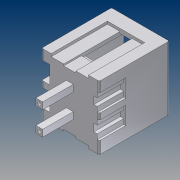
# Autodesk Inventor part: Wago Power In
Saved by Autodesk Inventor 2012 (Build 160160000, 160)
## iProperties
Category: PARTsolutions
Company: Team 801
Created: 2007-11-01
Part Number: Wago Power In
Catalog Web Link: www.team801.org
Description: 734-132 TO 734-154 - HEADER STRAIGHT SOLDER PIN. 1X1 MM / 0.039X 0.039 IN PIN SPACING 3.5 MM / 0.138 IN
Document SubType Name: Modeling
Designer: Jeffrey M
Mass: 0.424756 g
Surface Area: 9.45096 cm^2
Volume: 0.424756 cm^3
Density: 1 g/cm^3
Material: Default
NB: 734-132
NN: 734-132 TO 734-154
NT: HEADER STRAIGHT SOLDER PIN. 1X1 MM / 0.039X 0.039 IN PIN SPACING 3.5 MM / 0.138 IN
NBSYN: $BESTNR.
LINA: 734-132
BESTNR: 734-132
SPANNUNG: 250
BEMESSSTOSSSPG: 3
VERSCHMUTZGRAD: 2
STROM: 10
RM: 3.50
P: 2
HOEHE: 10.30
BREITE: 9.40
TIEFE: 8.50
FARBE: lichtgrau
GEWICHT: 0.602
EAN: 4017332322119
BEMERKUNGEN: L = (No. of poles - 1) x Pin Spacing + 5,9 mm
BOHRLOCHDURCHM: 1,4 +0,1 mm
RGB: 0.82,0.82,0.82,0
KT: DUMMY
PSOL_IDENT_0: {\\partserver001.servicenet\dplatte\cadenas\23d-libs\wago\pg03\serie734\0734-0132_0999-0962.prj},169
PSOL_IDENT_1: {VTYP=3D},{NB=734-132},{LINA=734-132},{NN=734-132 TO 734-154},{DATE=19.07.2007 11:20:09},{GEOMDATE=
PSOL_IDENT_2: 19.07.2007 00:00:00},{VERSION=},{LINEID=220},{LINESUBID=-1},{WBVAR=}  {NB=734-132},{LINA=734-132},{K
PSOL_IDENT_3: T=DUMMY},{BESTNR=734-132},{SPANNUNG=250},{BEMESSSTOSSSPG=3},{VERSCHMUTZGRAD=2},{STROM=10},{RM=3.50},
PSOL_IDENT_4: {P=2},{HOEHE=10.30},{BREITE=9.40},{TIEFE=8.50},{FARBE=lichtgrau},{GEWICHT=0.602},{EAN=4017332322119}
PSOL_IDENT_5: ,{BEMERKUNGEN=L = (No. of poles - 1) x Pin Spacing + 5,9 mm},{BOHRLOCHDURCHM=1,4 +0,1 mm},{RGB=0.82,
PSOL_IDENT_6: 0.82,0.82,0}
Title: Wago Power In
Author: Jeffrey M
Comments: HEADER STRAIGHT SOLDER PIN. 1X1 MM / 0.039X 0.039 IN PIN SPACING 3.5 MM / 0.138 IN
Autodesk Inventor part; units mm, degrees
ref_plane "YZ Plane" through (0, 0, 0) normal (1, 0, 0) x (0, 1, 0)
ref_plane "XZ Plane" through (0, 0, 0) normal (0, 1, 0) x (-1, 0, 0)
ref_plane "XY Plane" through (0, 0, 0) normal (0, 0, 1) x (1, 0, 0)
sketch "Skizze_1" plane through (0, 0, 0) normal (0, 0, 1) x (1, 0, 0)
  arc A0 (-4.15, 0.2) -> (-3.95, 0) centre (-3.95, 0.2) ccw
  line L0 (-3.95, 0) -> (4.15, 0)
  arc A1 (4.15, 0) -> (4.35, 0.2) centre (4.15, 0.2) ccw
  line L1 (4.35, 0.2) -> (4.35, 10.1)
  arc A2 (4.35, 10.1) -> (4.15, 10.3) centre (4.15, 10.1) ccw
  line L2 (4.15, 10.3) -> (-3.95, 10.3)
  arc A3 (-3.95, 10.3) -> (-4.15, 10.1) centre (-3.95, 10.1) ccw
  line L3 (-4.15, 10.1) -> (-4.15, 0.2)
  constraints: 8 end point, 8 point on circle, 4 centre point
extrude "Extrusion1" add sketch "Skizze_1" along normal blind 9.4
sketch "Skizze_2" plane through (0, 0, 0.95) normal (0, 0, 1) x (1, 0, 0)
  line L0 (-2.35, 10.3) -> (-2.35, 2.6)
  line L1 (-2.35, 2.6) -> (2.35, 2.6)
  line L2 (2.35, 2.6) -> (2.35, 10.3)
  line L3 (2.35, 10.3) -> (-2.35, 10.3)
  constraints: 8 end point
extrude "Extrusion2" cut sketch "Skizze_2" along normal blind 7.5
sketch "Skizze_3" plane through (0, 10.3, 0) normal (0, 1, 0) x (1, 0, 0)
  line L0 (-0.9, -0.95) -> (0.9, -0.95)
  line L1 (0.9, -0.95) -> (0.9, -0.65)
  line L2 (0.9, -0.65) -> (-0.9, -0.65)
  line L3 (-0.9, -0.65) -> (-0.9, -0.95)
  constraints: 8 end point
extrude "Extrusion3" cut sketch "Skizze_3" against normal blind 7.7
sketch "Skizze_4" plane through (0, 10.3, 0) normal (0, 1, 0) x (1, 0, 0)
  line L0 (-0.9, -8.45) -> (-0.9, -8.75)
  line L1 (-0.9, -8.75) -> (0.9, -8.75)
  line L2 (0.9, -8.75) -> (0.9, -8.45)
  line L3 (0.9, -8.45) -> (-0.9, -8.45)
  constraints: 8 end point
extrude "Extrusion4" cut sketch "Skizze_4" against normal blind 7.7
sketch "Skizze_5" plane through (0, 10.3, 0) normal (0, 1, 0) x (1, 0, 0)
  line L0 (2.35, -0.95) -> (2.35, -2.9)
  line L1 (2.35, -2.9) -> (3.95, -2.9)
  line L2 (3.95, -2.9) -> (3.95, -0.95)
  line L3 (3.95, -0.95) -> (2.35, -0.95)
  constraints: 8 end point
extrude "Extrusion5" cut sketch "Skizze_5" against normal blind 6
sketch "Skizze_6" plane through (0, 10.3, 0) normal (0, 1, 0) x (1, 0, 0)
  line L0 (2.35, -6.7) -> (3.95, -6.7)
  line L1 (3.95, -6.7) -> (3.95, -4.75)
  line L2 (3.95, -4.75) -> (2.35, -4.75)
  line L3 (2.35, -4.75) -> (2.35, -6.7)
  constraints: 8 end point
extrude "Extrusion6" cut sketch "Skizze_6" against normal blind 6
sketch "Skizze_7" plane through (0, 0, 0) normal (0, 1, 0) x (-1, 0, 0)
  line L0 (1.4, 1.7) -> (1.4, 4.5)
  line L1 (1.4, 4.5) -> (-1.4, 4.5)
  line L2 (-1.4, 4.5) -> (-1.4, 1.7)
  line L3 (-1.4, 1.7) -> (1.4, 1.7)
  constraints: 8 end point
extrude "Extrusion7" add sketch "Skizze_7" along normal blind 3.6
pattern_linear "Rectangular Pattern1" count 2 spacing 3.5 along (0, 0, 1) of "Extrusion7"
sketch "Skizze_9" plane through (0, 0, 0) normal (0, 1, 0) x (-1, 0, 0)
  line L0 (0.5, 2.6) -> (0.5, 3.6)
  line L1 (0.5, 3.6) -> (-0.5, 3.6)
  line L2 (-0.5, 3.6) -> (-0.5, 2.6)
  line L3 (-0.5, 2.6) -> (0.5, 2.6)
  constraints: 8 end point
extrude "Extrusion8" add sketch "Skizze_9" along normal blind 9.3
pattern_linear "Rectangular Pattern2" count 2 spacing 3.5 along (0, 0, 1) of "Extrusion8"
sketch "Skizze_11" plane through (0, 0, 0) normal (0, 1, 0) x (-1, 0, 0)
  line L0 (0.5, 2.6) -> (0.5, 3.6)
  line L1 (0.5, 3.6) -> (-0.5, 3.6)
  line L2 (-0.5, 3.6) -> (-0.5, 2.6)
  line L3 (-0.5, 2.6) -> (0.5, 2.6)
  constraints: 8 end point
extrude "Extrusion9" add sketch "Skizze_11" against normal blind 4.5
pattern_linear "Rectangular Pattern3" count 2 spacing 3.5 along (0, 0, 1) of "Extrusion9"
sketch "Skizze_13" plane through (0, 0, 0) normal (0, 1, 0) x (-1, 0, 0)
  line L0 (2.75, 0) -> (2.75, 0.4)
  line L1 (2.75, 0.4) -> (0.9, 0.4)
  line L2 (0.9, 0.4) -> (0.9, 0.65)
  line L3 (0.9, 0.65) -> (-0.9, 0.65)
  line L4 (-0.9, 0.65) -> (-0.9, 0.4)
  line L5 (-0.9, 0.4) -> (-2.75, 0.4)
  line L6 (-2.75, 0.4) -> (-2.75, 0)
  line L7 (-2.75, 0) -> (2.75, 0)
  constraints: 16 end point
extrude "Extrusion10" cut sketch "Skizze_13" along normal blind 8.3
sketch "Skizze_14" plane through (0, 0, 0) normal (0, 1, 0) x (-1, 0, 0)
  line L0 (2.75, 9.4) -> (-2.75, 9.4)
  line L1 (-2.75, 9.4) -> (-2.75, 9)
  line L2 (-2.75, 9) -> (-0.9, 9)
  line L3 (-0.9, 9) -> (-0.9, 8.75)
  line L4 (-0.9, 8.75) -> (0.9, 8.75)
  line L5 (0.9, 8.75) -> (0.9, 9)
  line L6 (0.9, 9) -> (2.75, 9)
  line L7 (2.75, 9) -> (2.75, 9.4)
  constraints: 16 end point
extrude "Extrusion11" cut sketch "Skizze_14" along normal blind 8.3
sketch "Skizze_15" plane through (0, 0, 0) normal (0, 1, 0) x (-1, 0, 0)
  line L0 (4.15, 1.8) -> (4.15, 4.4)
  line L1 (4.15, 4.4) -> (2.95, 4.4)
  line L2 (2.95, 4.4) -> (2.95, 1.8)
  line L3 (2.95, 1.8) -> (4.15, 1.8)
  constraints: 8 end point
extrude "Extrusion12" cut sketch "Skizze_15" along normal blind 9.15
pattern_linear "Rectangular Pattern4" count 2 spacing 3.5 along (0, 0, 1) of "Extrusion12"
sketch "Skizze_17" plane through (0, 0, 0) normal (0, 1, 0) x (-1, 0, 0)
  line L0 (-3.55, 2.55) -> (-3.55, 3.65)
  line L1 (-3.55, 3.65) -> (-4.05, 3.65)
  line L2 (-4.05, 3.65) -> (-4.05, 4.4)
  line L3 (-4.05, 4.4) -> (-4.35, 4.4)
  line L4 (-4.35, 4.4) -> (-4.35, 1.8)
  line L5 (-4.35, 1.8) -> (-4.05, 1.8)
  line L6 (-4.05, 1.8) -> (-4.05, 2.55)
  line L7 (-4.05, 2.55) -> (-3.55, 2.55)
  constraints: 16 end point
extrude "Extrusion13" cut sketch "Skizze_17" along normal blind 3.9
sketch "Skizze_18" plane through (0, 0, 0) normal (0, 1, 0) x (-1, 0, 0)
  line L0 (-3.55, 6.05) -> (-3.55, 7.15)
  line L1 (-3.55, 7.15) -> (-4.05, 7.15)
  line L2 (-4.05, 7.15) -> (-4.05, 7.9)
  line L3 (-4.05, 7.9) -> (-4.35, 7.9)
  line L4 (-4.35, 7.9) -> (-4.35, 5.3)
  line L5 (-4.35, 5.3) -> (-4.05, 5.3)
  line L6 (-4.05, 5.3) -> (-4.05, 6.05)
  line L7 (-4.05, 6.05) -> (-3.55, 6.05)
  constraints: 16 end point
extrude "Extrusion14" cut sketch "Skizze_18" along normal blind 3.9
sketch "Sketch15" plane through (-0.5, 9.3, 6.1) normal (0, 1, 0) x (1, 0, 0)
  line L0 (0, 0) -> (1, 0) projected
  line L1 (0, -1) -> (0, 0) projected
  line L2 (1, -1) -> (0, -1) projected
  line L3 (1, 0) -> (1, -1) projected
  line L4 (0, -1) -> (1, 0) construction
  point P0 (0.5, 6.1)
  point P1 (0.5, -0.5)
  constraints: 2 end point, 1 midpoint
sketch "Sketch16" plane through (-0.5, 9.3, 6.1) normal (0, 1, 0) x (1, 0, 0)
  line L0 (0, 3.5) -> (1, 3.5) construction
  line L1 (0, 2.5) -> (0, 3.5) construction
  line L2 (1, 2.5) -> (0, 2.5) construction
  line L3 (1, 3.5) -> (1, 2.5) construction
  line L4 (0, 0) -> (1, 0) construction
  line L5 (0, -1) -> (0, 0) construction
  line L6 (1, -1) -> (0, -1) construction
  line L7 (1, 0) -> (1, -1) construction
  line L8 (1, -1) -> (0, 0) construction
  line L9 (1, 2.5) -> (0, 3.5) construction
  circle A0 centre (0.5, 3) radius 0.25
  circle A1 centre (0.5, -0.5) radius 0.25
  point P0 (0.5, 6.1)
  dimension "d52" = 0.5
  constraints: 4 end point, 2 centre point, 2 midpoint, 1 equal radius, 1 parallel
  measures "d52" diameter of A0
extrude "Extrusion15" cut sketch "Sketch16" against normal through all
body "Solid1"
